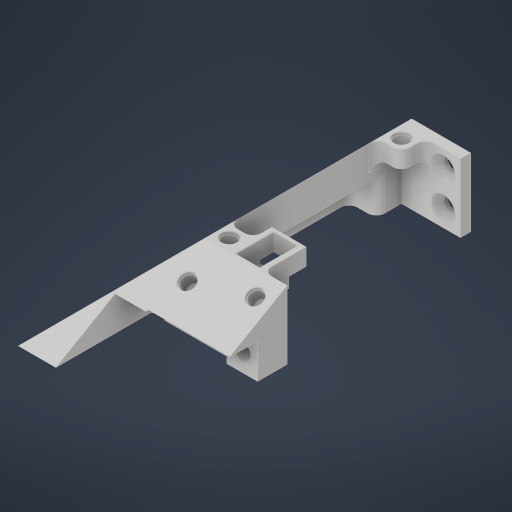
# Autodesk Inventor part: MocowanieCzujnikaBezScianki
Saved by Autodesk Inventor 2023 (Build 270158000, 158)
## iProperties
Created: 2021-11-14
Part Number: MocowanieCzujnikaBezScianki
Material: Ogólny
Document SubType Name: Modeling
Designer: Michał
Density: 1 g/cm^3
Appearance: Domyślna
Author: Michał
Autodesk Inventor part; units mm, degrees
ref_plane "YZ Plane" through (0, 0, 0) normal (1, 0, 0) x (0, 1, 0)
ref_plane "XZ Plane" through (0, 0, 0) normal (0, 1, 0) x (-1, 0, 0)
ref_plane "XY Plane" through (0, 0, 0) normal (0, 0, 1) x (1, 0, 0)
sketch "Szkic1" plane through (0, 0, 0) normal (0, 1, 0) x (-1, 0, 0)
  line L0 (0, 0) -> (20, 0)
  line L1 (20, 0) -> (20, -95)
  line L2 (20, -95) -> (0, -95)
  line L3 (0, -95) -> (0, 0)
  dimension "d0" = 95
  dimension "d1" = 20
  constraints: 8 end point, 2 parallel, 1 horizontal, 1 perpendicular
  measures "d0" distance of L2.end L0.start
  measures "d1" distance between parallel lines of L3 L1
extrude "Wyciągnięcie proste1" add sketch "Szkic1" along normal blind 20
sketch "Szkic2" plane through (-20, 0, 0) normal (0, 0, 1) x (1, 0, 0)
  line L0 (20, 0) -> (20, 20) projected
  line L1 (20, 0) -> (20, 20)
  line L2 (20, 20) -> (0, 20)
  line L3 (0, 20) -> (20, 20) projected
  line L4 (20, 0) -> (0, 0) projected
  line L5 (20, 0) -> (0, 20)
  dimension "d4" = 45
  constraints: 6 end point, 1 collinear, 1 point on line
  measures "d4" angle of L0 L5
extrude "Wyciągnięcie proste2" cut sketch "Szkic2" against normal up to next
sketch "Szkic3" plane through (-20, 0, -95) normal (-1, 0, 0) x (0, 0, 1)
  line L0 (95, 0) -> (0, 0) projected
  line L1 (95, 0) -> (95, 20) projected
  line L2 (95, 0) -> (95, 20)
  line L3 (95, 20) -> (60.359, 20)
  line L4 (0, 20) -> (95, 20) projected
  line L5 (95, 0) -> (60.359, 20)
  dimension "d7" = 30
  constraints: 6 end point, 1 point on line, 1 vertical
  measures "d7" angle of L3 L5
extrude "Wyciągnięcie proste3" cut sketch "Szkic3" against normal up to next
sketch "Szkic4" plane through (-20, 0, -95) normal (-1, 0, 0) x (0, 0, 1)
  line L0 (0, 20) -> (60.359, 20) projected
  line L1 (60.359, 20) -> (60.359, 0)
  line L2 (95, 0) -> (60.359, 20) construction
  line L3 (60.359, 20) -> (95, 0) construction
  line L4 (95, 0) -> (60.359, 0) construction
  line L5 (77.6795, 10) -> (77.6795, 0) construction
  line L6 (0, 0) -> (95, 0) construction
  line L7 (77.6795, 10) -> (68.6795, 10) construction
  line L8 (68.6795, 10) -> (68.6795, 0)
  line L9 (60.359, 0) -> (68.6795, 0)
  line L10 (68.6795, 10) -> (60.359, 10)
  line L11 (68.6795, 10) -> (60.359, 20)
  dimension "d11" = 10
  dimension "d12" = 9
  constraints: 18 end point, 2 collinear, 2 horizontal, 2 midpoint, 2 perpendicular, 2 point on line, 1 vertical
  measures "d11" distance of L5.start L5.end
  measures "d12" distance of L5.start L7.end
extrude "Wyciągnięcie proste4" add sketch "Szkic4" along normal blind 24
sketch "Szkic5" plane through (-20, 0, -26.3205) normal (0, 0, 1) x (1, 0, 0)
  line L0 (-24, 0) -> (-15, 0) construction
  line L1 (0, 0) -> (-24, 0) projected
  line L2 (-15, 0) -> (9, 0) construction
  line L3 (0, 0) -> (20, 0) construction
  line L4 (9, 0) -> (9, 10)
  line L5 (9, 10) -> (-15, 10)
  line L6 (0, 10) -> (-24, 10) construction
  line L7 (-15, 0) -> (-15, 10)
  line L8 (-15, 0) -> (9, 0)
  dimension "d15" = 9
  dimension "d16" = 24
  dimension "d17" = 10
  constraints: 12 end point, 3 point on line, 2 perpendicular, 1 collinear
  measures "d15" distance of L0.start L0.end
  measures "d16" distance of L0.end L2.end
  measures "d17" distance of L2.end L4.end
extrude "Wyciągnięcie proste5" cut sketch "Szkic5" against normal blind 1.5 and the other way blind 100
sketch "Szkic6" plane through (-20, 0, -95) normal (-1, 0, 0) x (0, 0, 1)
  line L0 (0, 20) -> (0, 0) projected
  line L1 (0, 0) -> (95, 0) projected
  line L2 (0, 20) -> (3, 20)
  line L3 (3, 20) -> (3, 0)
  line L4 (3, 0) -> (0, 0)
  line L5 (0, 0) -> (0, 20)
  dimension "d22" = 3
  constraints: 8 end point, 2 parallel, 1 horizontal, 1 perpendicular, 1 point on line
  measures "d22" distance between parallel lines of L3 L0
extrude "Wyciągnięcie proste6" add sketch "Szkic6" along normal blind 17.26
sketch "Szkic7" plane through (-44, 0, -95) normal (-1, 0, 0) x (0, 0, 1)
  line L0 (60.359, 0) -> (68.6795, 0) projected
  line L1 (68.6795, 0) -> (69.0287, 0)
  line L2 (95, 0) -> (67.1795, 0) projected
  line L3 (68.6795, 0) -> (68.6795, 10) projected
  line L4 (68.6795, 10) -> (69.0287, 0)
  line L5 (60.359, 20) -> (68.6795, 10) projected
  line L6 (68.6795, 0) -> (68.6795, 10)
  dimension "d25" = 88
  constraints: 6 end point, 1 perpendicular, 1 point on line
  measures "d25" angle of L4 L1
extrude "Wyciągnięcie proste7" add sketch "Szkic7" against normal up to surface (9 mm away)
sketch "Szkic8" plane through (0, 0, 0) normal (0, -1, 0) x (1, 0, 0)
  line L0 (0, -95) -> (0, 0) construction
  line L1 (0, -95) -> (0, -30) construction
  line L2 (0, -30) -> (-9.26, -30) construction
  line L3 (0, -95) -> (0, -90) construction
  line L4 (0, -90) -> (-9.26, -90) construction
  dimension "d28" = 65
  dimension "d29" = 9.26
  dimension "d30" = 5
  dimension "d31" = 9.26
  constraints: 8 end point, 2 coincident, 2 perpendicular, 2 point on line
  measures "d28" distance of L0.start L1.end
  measures "d29" distance of L1.end L2.end
  measures "d30" distance of L0.start L3.end
  measures "d31" distance of L3.end L4.end
hole "Otwór1" at (-9.26, 0, -90) at (-9.26, 0, -30) direction (0, 1, 0) diameter 4.134 depth 7 thread size "M5x0.8" class "6H" standard "ISO Metric profile"
sketch "Szkic9" plane through (0, 0, 0) normal (0, -1, 0) x (1, 0, 0)
  line L0 (-11, -27.8205) -> (-35, -27.8205) projected
  line L1 (-15, -27.8205) -> (-11, -27.8205)
  circle A0 centre (-9.26, -30) radius 2.067 projected
  circle A1 centre (-9.26, -30) radius 2.7889
  line L2 (-20, -34.641) -> (0, 0) projected
  line L3 (-15, -27.8205) -> (-20, -34.641)
  line L4 (-12.0489, -30) -> (-12.0489, -84.641)
  line L5 (-12.0489, -84.641) -> (-20, -84.641)
  line L6 (-20, -92) -> (-20, -34.641) projected
  line L7 (-20, -84.641) -> (-20, -34.641)
  dimension "d72" = 4
  dimension "d73" = 50
  constraints: 10 end point, 2 collinear, 2 point on circle, 1 centre point, 1 coincident, 1 perpendicular, 1 point on line, 1 tangent, 1 vertical
  measures "d72" distance of L1.start L0.start
  measures "d73" distance of L2.start L5.end
extrude "Wyciągnięcie proste8" cut sketch "Szkic9" against normal up to surface (10 mm away) contours A1 L4 L5 L6 L3 L0
sketch "Szkic11" plane through (-44, 0, -95) normal (-1, 0, 0) x (0, 0, 1)
  line L0 (60.359, 20) -> (95, 0) projected
  line L1 (60.359, 20) -> (68.6795, 10) projected
  line L2 (60.359, 20) -> (68.6795, 10)
  line L3 (68.6795, 10) -> (77.6795, 10) projected
  line L4 (68.6795, 10) -> (77.1662, 10.2964)
  line L5 (60.359, 20) -> (77.1662, 10.2964)
  line L6 (69.0287, 0) -> (68.6795, 10) projected
  dimension "d42" = 90
  constraints: 6 end point, 2 collinear, 1 point on line
  measures "d42" angle of L6 L4
extrude "Wyciągnięcie proste9" add sketch "Szkic11" against normal up to next contours L0 L4 L1
sketch "Szkic12" plane through (-20, 0, -92) normal (-1, 0, 0) x (0, 0, 1)
  line L0 (57.359, 10) -> (57.359, 20) projected
  line L1 (57.359, 20) -> (50.359, 20)
  line L2 (50.359, 20) -> (50.359, 15)
  line L3 (50.359, 15) -> (57.359, 15)
  line L4 (57.359, 15) -> (57.359, 20)
  line L5 (0, 20) -> (0, 0) projected
  line L6 (0, 20) -> (7, 20)
  line L7 (7, 20) -> (7, 15)
  line L8 (7, 15) -> (0, 15)
  line L9 (0, 15) -> (0, 20)
  point P0 (92, 0)
  dimension "d45" = 5
  dimension "d46" = 7
  constraints: 16 end point, 4 parallel, 2 equal length, 2 horizontal, 2 perpendicular
  measures "d45" distance between parallel lines of L1 L3
  measures "d46" distance between parallel lines of L0 L2
extrude "Wyciągnięcie proste10" add sketch "Szkic12" along normal blind 7
sketch "Szkic13" plane through (-27, 20, -41.641) normal (0, 1, 0) x (1, 0, 0)
  line L0 (0, -7) -> (0, 0) construction
  line L1 (0, -3.5) -> (3.5, -3.5) construction
  line L2 (3.5, -3.5) -> (7, -3.5) construction
  line L3 (7, -15.3205) -> (7, -24.3205) construction
  line L4 (3.5, -3.5) -> (3.5, 0) construction
  line L5 (0, 50.359) -> (0, 43.359) construction
  line L6 (0, 46.859) -> (3.5, 46.859) construction
  line L7 (3.5, 46.859) -> (7, 46.859) construction
  line L8 (7, 53.359) -> (7, 43.359) construction
  line L9 (7, 43.359) -> (0, 43.359) construction
  line L10 (3.5, 46.859) -> (3.5, 43.359) construction
  point P0 (27, -41.641)
  point P1 (7, -2.0649)
  point P2 (7, -7)
  constraints: 12 end point, 4 point on line, 3 equal length, 3 midpoint, 1 horizontal, 1 perpendicular, 1 vertical
hole "Otwór2" at (-23.5, 20, -38.141) at (-23.5, 20, -88.5) direction (0, -1, 0) diameter 4 depth 4 counterbore diameter 4.5 counterbore depth 0.6
sketch "Szkic14" plane through (-37.26, 0, -92) normal (0, 0, 1) x (1, 0, 0)
  line L0 (0, 0) -> (0, 20) construction
  line L1 (0, 15) -> (5, 15) construction
  line L2 (5, 15) -> (5, 20) construction
  line L3 (10.26, 20) -> (0, 20) construction
  line L4 (0, 5) -> (5, 5) construction
  line L5 (5, 5) -> (5, 0) construction
  line L6 (0, 0) -> (37.26, 0) construction
  dimension "d56" = 5
  dimension "d57" = 5
  dimension "d58" = 5
  constraints: 8 end point, 4 point on line, 2 horizontal, 2 perpendicular, 1 parallel
  measures "d56" distance of L1.start L1.end
  measures "d57" distance of L1.end L2.end
  measures "d58" distance of L4.end L5.end
hole "Otwór3" at (-32.26, 15, -92) at (-32.26, 5, -92) direction (0, 0, -1) diameter 3.4 end through all countersink diameter 6.9 countersink angle 84.225
ref_plane "Płaszczyzna konstrukcyjna1" through (8, -8, -95) normal (0, -1, 0) x (1, 0, 0)
sketch "Szkic17" plane through (-20, 0, -27.8205) normal (0, 0, 1) x (1, 0, 0)
  line L0 (0, 0) -> (0, 5) construction
  circle A0 centre (0, 5) radius 2.5
  line L1 (0, 5) -> (-6, 5) construction
  line L2 (-6, 5) -> (-12, 5) construction
  circle A1 centre (-6, 5) radius 2.5
  circle A2 centre (-12, 5) radius 2.5
  line L3 (0, 0) -> (5, 0) construction
  line L4 (0, 0) -> (5, 0)
  point P0 (20, 0)
  dimension "d75" = 5
  dimension "d76" = 5
  dimension "d77" = 6
  dimension "d81" = 5
  constraints: 8 end point, 3 centre point, 3 coincident, 2 equal radius, 2 horizontal, 1 collinear, 1 point on line, 1 vertical
  measures "d75" distance of L0.start L0.end
  measures "d76" diameter of A0
  measures "d77" distance of L1.start L1.end
  measures "d81" distance of L0.start L3.end
extrude "Wyciągnięcie proste13" cut sketch "Szkic17" against normal up to next
sketch "Szkic18" plane through (-44, 0, -25.9713) normal (0, 0.0348995, 0.9993908) x (1, 0, 0)
  line L0 (0, 0) -> (9, 0) construction
  line L1 (0, 0) -> (4.5, 0) construction
  line L2 (4.5, 0) -> (4.5, 5.25) construction
  point P0 (44, -0.9064)
  dimension "d84" = 4.5
  dimension "d85" = 5.25
  constraints: 4 end point, 1 coincident, 1 midpoint, 1 perpendicular
  measures "d84" distance of L0.start L1.end
  measures "d85" distance of L1.end L2.end
hole "Otwór4" at (-39.5, 5.2468, -26.1545) direction (0, -0.0348995, -0.9993908) diameter 4 depth 4 counterbore diameter 4.5 counterbore depth 0.6
sketch "Szkic19" plane through (-20, 10, -17.3205) normal (0, 0.8660254, 0.5) x (1, 0, 0)
  line L0 (-7, 20) -> (-24, 20) projected
  line L1 (-24, 20) -> (-19.5, 20)
  line L2 (-19.5, 20) -> (-19.5, 14.4)
  line L3 (-3.5, 20) -> (-3.5, 10)
  line L4 (0, 10) -> (-24, 10) projected
  line L5 (20, -20) -> (0, 20) construction
  line L6 (0, 20) -> (20, -20) construction
  line L7 (-3.5, 20) -> (0, 20) construction
  dimension "d93" = 4.5
  dimension "d94" = 5.6
  dimension "d117" = 10
  dimension "d118" = 3.5
  constraints: 10 end point, 2 point on line, 1 horizontal, 1 parallel, 1 vertical
  measures "d93" distance of L0.end L1.end
  measures "d94" distance of L1.end L2.end
  measures "d117" distance of L3.start L3.end
  measures "d118" distance of L3.start L6.start
hole "Otwór5" at (-23.5, 15, -25.9808) at (-39.5, 17.2, -29.7913) direction (0, -0.8660254, -0.5) diameter 4 depth 4 counterbore diameter 4.5 counterbore depth 0.6
mirror "Odbij1" about plane through (-44, 14.0631, -26.7232) normal (-1, 0, 0) remove original yes
sketch "Szkic20" plane through (-61, 15, -34.641) normal (1, 0, 0) x (0, 0, -1)
  line L0 (0, 5) -> (-34.641, -15) projected
  line L1 (0, 5) -> (12.5, 5)
  line L2 (12.5, 5) -> (12.5, 0)
  line L3 (12.5, 0) -> (0, 0)
  line L4 (0, 0) -> (0, 5)
  dimension "d119" = 12.5
  dimension "d120" = 5
  constraints: 8 end point, 2 parallel, 1 horizontal, 1 perpendicular
  measures "d119" distance of L2.end L3.end
  measures "d120" distance of L1.end L2.end
extrude "Wyciągnięcie proste14" add sketch "Szkic20" along normal blind 10
sketch "Szkic21" plane through (-51, 15, -34.641) normal (1, 0, 0) x (0, 0, -1)
  line L0 (0, 5) -> (0, -15) construction
  line L1 (0, 5) -> (4.5, 5) construction
  line L2 (5.75, 5) -> (1.25, 5) construction
  line L3 (4.5, 5) -> (7.5, 5)
  line L4 (7.5, 5) -> (7.5, -3)
  line L5 (7.5, -3) -> (4.5, -3)
  line L6 (4.5, -3) -> (4.5, 5)
  point P0 (-34.641, -15)
  dimension "d107" = 4.5
  dimension "d108" = 3
  dimension "d109" = 8
  constraints: 10 end point, 2 parallel, 1 horizontal, 1 perpendicular, 1 point on line
  measures "d107" distance of L0.start L1.end
  measures "d108" distance between parallel lines of L4 L6
  measures "d109" distance between parallel lines of L5 L3
extrude "Wyciągnięcie proste15" add sketch "Szkic21" against normal up to surface (10 mm away)
sketch "Szkic22" plane through (-70.83, 20, -95) normal (0, 1, 0) x (1, 0, 0)
  line L0 (18.33, -48.859) -> (11.33, -48.859)
  line L1 (11.33, -48.859) -> (11.33, -59.859)
  line L2 (11.33, -59.859) -> (18.33, -59.859)
  line L3 (18.33, -59.859) -> (18.33, -48.859)
  line L4 (18.33, -48.859) -> (19.83, -48.859) construction
  line L5 (19.83, -47.859) -> (19.83, -60.3354) construction
  line L6 (19.83, -47.859) -> (19.83, -60.359) construction
  line L7 (11.33, -48.859) -> (9.83, -48.859) construction
  line L8 (9.83, -47.859) -> (19.83, -47.859) projected
  line L9 (9.83, -47.859) -> (9.83, -53.359) construction
  line L10 (9.83, -53.359) -> (9.83, -47.859) construction
  point P0 (70.83, -95)
  dimension "d114" = 7
  dimension "d123" = 11
  dimension "d124" = 1
  constraints: 16 end point, 2 collinear, 2 parallel, 2 perpendicular, 2 point on line, 2 vertical, 1 horizontal
  measures "d114" distance of L0.start L0.end
  measures "d123" distance of L2.end L0.start
  measures "d124" distance between parallel lines of L8 L0
extrude "Wyciągnięcie proste16" cut sketch "Szkic22" against normal blind 6
sketch "Szkic23" plane through (-88, 0, -95) normal (-0.7071068, 0.7071068, 0) x (-0.7071068, -0.7071068, 0)
  line L0 (-28.2843, 10) -> (-28.2843, 53.359) projected
  line L1 (-36.7696, 60.359) -> (-24.7487, 60.359) projected
  point P0 (-18.6983, 49.895)
  point P1 (-9.6983, 29.895)
  dimension "d125" = 9.586
  dimension "d126" = 10.464
  dimension "d127" = 20
  dimension "d128" = 18.586
  measures "d125" distance from line of L0 point (-18.698, 49.895)
  measures "d126" distance from line of L1 point (-18.698, 49.895)
  measures "d127" vertical distance of point (-9.698, 29.895) point (-18.698, 49.895)
  measures "d128" distance from line of L0 point (-9.698, 29.895)
hole "Otwór6" at (-74.7783, 13.2217, -45.105) at (-81.1423, 6.8577, -65.105) direction (0.7071068, -0.7071068, 0) diameter 4 depth 4 counterbore diameter 4.5 counterbore depth 0.6
fillet "Fillet1" radius 2.5 14 edges at (-64.5, 15, -92) (-68, 15, -88.5) (-61, 17.5, -85) (-68, 17.5, -85) (-61, 17.5, -92) (-75.9511, 5, -84.641) (-68, 5, -84.641) (-76.227, 10, -28.7906) (-75.9511, 10, -57.3205) (-68, 17.5, -41.641) (-61, 17.5, -41.641) (-51, 17.5, -34.641) (-59.5, 15, -34.641) (-68, 15, -38.141)
